Autodesk Fusion 360 part; units mm, degrees
(part 2 of 3)
  spline S416 degree 2 poles (1.0498, 18.6064) (0.9543, 18.5109) (0.9543, 18.3438) knots 0 0 0 1 1 1
  spline S417 degree 2 poles (1.3053, 18.7019) (1.1453, 18.7019) (1.0498, 18.6064) knots 0 0 0 1 1 1
  spline S418 degree 2 poles (1.5942, 18.5742) (1.4724, 18.7019) (1.3053, 18.7019) knots 0 0 0 1 1 1
  spline S419 degree 2 poles (1.7159, 18.2554) (1.7159, 18.4464) (1.5942, 18.5742) knots 0 0 0 1 1 1
  spline S420 degree 2 poles (1.704, 18.1289) (1.7159, 18.2101) (1.7159, 18.2554) knots 0 0 0 1 1 1
  line L121 (2.3987, 18.0788) -> (1.704, 18.1289)
  spline S421 degree 2 poles (2.3414, 18.3939) (2.3414, 18.2793) (2.3987, 18.0788) knots 0 0 0 1 1 1
  spline S422 degree 2 poles (2.4751, 18.7341) (2.3414, 18.6088) (2.3414, 18.3939) knots 0 0 0 1 1 1
  spline S423 degree 2 poles (2.8524, 18.8595) (2.6088, 18.8595) (2.4751, 18.7341) knots 0 0 0 1 1 1
  spline S424 degree 2 poles (3.2344, 18.7293) (3.0911, 18.8595) (2.8524, 18.8595) knots 0 0 0 1 1 1
  spline S425 degree 2 poles (3.3776, 18.4035) (3.3776, 18.5992) (3.2344, 18.7293) knots 0 0 0 1 1 1
  spline S426 degree 2 poles (3.2642, 18.0967) (3.3776, 18.2172) (3.3776, 18.4035) knots 0 0 0 1 1 1
  spline S427 degree 2 poles (2.8571, 17.9188) (3.1508, 17.9761) (3.2642, 18.0967) knots 0 0 0 1 1 1
  line L122 (2.9861, 16.9471) -> (2.8571, 17.9188)
  spline S428 degree 2 poles (3.5292, 17.2205) (3.3131, 17.0426) (2.9861, 16.9471) knots 0 0 0 1 1 1
  spline S429 degree 2 poles (3.8575, 17.6741) (3.7453, 17.3983) (3.5292, 17.2205) knots 0 0 0 1 1 1
  spline S430 degree 2 poles (3.9697, 18.4273) (3.9697, 17.9498) (3.8575, 17.6741) knots 0 0 0 1 1 1
  spline S431 degree 2 poles (3.8181, 19.2176) (3.9697, 18.9168) (3.9697, 18.4273) knots 0 0 0 1 1 1
  spline S432 degree 2 poles (3.386, 19.6783) (3.6665, 19.5184) (3.8181, 19.2176) knots 0 0 0 1 1 1
  spline S433 degree 2 poles (2.7998, 19.8383) (3.1054, 19.8383) (3.386, 19.6783) knots 0 0 0 1 1 1
  spline S434 degree 2 poles (2.3808, 19.7416) (2.5563, 19.8383) (2.7998, 19.8383) knots 0 0 0 1 1 1
  spline S435 degree 2 poles (2.0979, 19.4706) (2.2054, 19.6449) (2.3808, 19.7416) knots 0 0 0 1 1 1
  spline S436 degree 2 poles (1.9809, 19.1603) (2.0311, 19.3632) (2.0979, 19.4706) knots 0 0 0 1 1 1
  spline S437 degree 2 poles (1.6586, 19.5351) (1.8425, 19.411) (1.9809, 19.1603) knots 0 0 0 1 1 1
  spline S438 degree 2 poles (1.248, 19.6592) (1.4748, 19.6592) (1.6586, 19.5351) knots 0 0 0 1 1 1
  spline S439 degree 2 poles (0.6058, 19.3537) (0.8612, 19.6592) (1.248, 19.6592) knots 0 0 0 1 1 1
  spline S440 degree 2 poles (0.3503, 18.3629) (0.3503, 19.0481) (0.6058, 19.3537) knots 0 0 0 1 1 1
  spline S441 degree 2 poles (0.5843, 17.4401) (0.3503, 17.766) (0.3503, 18.3629) knots 0 0 0 1 1 1
  spline S442 degree 2 poles (1.2575, 16.9996) (0.8183, 17.1142) (0.5843, 17.4401) knots 0 0 0 1 1 1
  line L123 (1.4223, 17.9188) -> (1.2575, 16.9996)
  spline S443 degree 2 poles (1.0582, 18.0644) (1.162, 17.957) (1.4223, 17.9188) knots 0 0 0 1 1 1
  line L124 (6.5014, 21.9082) -> (6.5014, 20.9722)
  line L125 (6.5014, 20.9722) -> (5.3999, 21.9082)
  line L126 (5.3999, 21.9082) -> (6.5014, 21.9082)
  line L127 (7.91, 22.7558) -> (7.91, 21.9082)
  line L128 (7.2558, 22.7558) -> (7.91, 22.7558)
  line L129 (7.2558, 23.1951) -> (7.2558, 22.7558)
  line L130 (6.5014, 23.1951) -> (7.2558, 23.1951)
  line L131 (6.5014, 22.7558) -> (6.5014, 23.1951)
  line L132 (4.3503, 22.7558) -> (6.5014, 22.7558)
  line L133 (4.3503, 21.9082) -> (4.3503, 22.7558)
  line L134 (6.456, 20.1367) -> (4.3503, 21.9082)
  line L135 (7.2558, 20.1367) -> (6.456, 20.1367)
  line L136 (7.2558, 21.9082) -> (7.2558, 20.1367)
  line L137 (7.91, 21.9082) -> (7.2558, 21.9082)
  spline S444 degree 2 poles (2.1481, 21.2015) (1.4867, 21.2015) (1.242, 21.309) knots -1 -1 -1 0 0 0
  spline S445 degree 2 poles (1.242, 21.309) (0.9973, 21.4164) (0.9973, 21.6575) knots -1 -1 -1 0 0 0
  spline S446 degree 2 poles (0.9973, 21.6575) (0.9973, 21.8939) (1.2373, 22.0121) knots -1 -1 -1 0 0 0
  spline S447 degree 2 poles (1.2373, 22.0121) (1.4772, 22.1303) (2.1743, 22.1303) knots -1 -1 -1 0 0 0
  spline S448 degree 2 poles (2.1743, 22.1303) (2.6494, 22.1303) (2.8738, 22.0789) knots -1 -1 -1 0 0 0
  spline S449 degree 2 poles (2.8738, 22.0789) (3.0983, 22.0276) (3.2021, 21.919) knots -1 -1 -1 0 0 0
  spline S450 degree 2 poles (3.2021, 21.919) (3.306, 21.8103) (3.306, 21.6623) knots -1 -1 -1 0 0 0
  spline S451 degree 2 poles (3.306, 21.6623) (3.306, 21.4379) (3.0613, 21.3197) knots -1 -1 -1 0 0 0
  spline S452 degree 2 poles (3.0613, 21.3197) (2.8165, 21.2015) (2.1481, 21.2015) knots -1 -1 -1 0 0 0
  spline S453 degree 2 poles (3.4158, 20.5044) (3.2224, 20.3779) (2.887, 20.3074) knots 0 0 0 1 1 1
  spline S454 degree 2 poles (3.8288, 20.9509) (3.688, 20.6787) (3.4158, 20.5044) knots 0 0 0 1 1 1
  spline S455 degree 2 poles (3.9697, 21.6647) (3.9697, 21.223) (3.8288, 20.9509) knots 0 0 0 1 1 1
  spline S456 degree 2 poles (3.528, 22.7749) (3.9697, 22.4526) (3.9697, 21.6647) knots 0 0 0 1 1 1
  spline S457 degree 2 poles (2.1337, 23.0972) (3.0863, 23.0972) (3.528, 22.7749) knots 0 0 0 1 1 1
  spline S458 degree 2 poles (1.3172, 22.9993) (1.7088, 23.0972) (2.1337, 23.0972) knots 0 0 0 1 1 1
  spline S459 degree 2 poles (0.9579, 22.8668) (1.1119, 22.9492) (1.3172, 22.9993) knots 0 0 0 1 1 1
  spline S460 degree 2 poles (0.6643, 22.6412) (0.8039, 22.7844) (0.9579, 22.8668) knots 0 0 0 1 1 1
  spline S461 degree 2 poles (0.4375, 22.2711) (0.5246, 22.4979) (0.6643, 22.6412) knots 0 0 0 1 1 1
  spline S462 degree 2 poles (0.3503, 21.691) (0.3503, 22.0443) (0.4375, 22.2711) knots 0 0 0 1 1 1
  spline S463 degree 2 poles (0.749, 20.5963) (0.3503, 20.9556) (0.3503, 21.691) knots 0 0 0 1 1 1
  spline S464 degree 2 poles (2.1457, 20.237) (1.1477, 20.237) (0.749, 20.5963) knots 0 0 0 1 1 1
  spline S465 degree 2 poles (2.887, 20.3074) (2.5515, 20.237) (2.1457, 20.237) knots 0 0 0 1 1 1
  line L138 (-4.8826, 21.6074) -> (-4.8826, 23.1258)
  spline S466 degree 2 poles (-5.0951, 21.8402) (-5.0139, 21.7411) (-4.8826, 21.6074) knots 0 0 0 1 1 1
  spline S467 degree 2 poles (-5.3792, 22.2329) (-5.1763, 21.9393) (-5.0951, 21.8402) knots 0 0 0 1 1 1
  spline S468 degree 2 poles (-6.0191, 22.9145) (-5.7278, 22.7271) (-5.3792, 22.2329) knots 0 0 0 1 1 1
  spline S469 degree 2 poles (-6.6302, 23.1019) (-6.3103, 23.1019) (-6.0191, 22.9145) knots 0 0 0 1 1 1
  spline S470 degree 2 poles (-7.1734, 22.9384) (-6.9311, 23.1019) (-6.6302, 23.1019) knots 0 0 0 1 1 1
  spline S471 degree 2 poles (-7.5327, 22.4896) (-7.4157, 22.7749) (-7.1734, 22.9384) knots 0 0 0 1 1 1
  spline S472 degree 2 poles (-7.6497, 21.691) (-7.6497, 22.2043) (-7.5327, 22.4896) knots 0 0 0 1 1 1
  spline S473 degree 2 poles (-7.5267, 20.921) (-7.6497, 21.1992) (-7.6497, 21.691) knots 0 0 0 1 1 1
  spline S474 degree 2 poles (-7.1734, 20.4901) (-7.4038, 20.6429) (-7.5267, 20.921) knots 0 0 0 1 1 1
  spline S475 degree 2 poles (-6.5324, 20.28) (-6.943, 20.3373) (-7.1734, 20.4901) knots 0 0 0 1 1 1
  line L139 (-6.4536, 21.2541) -> (-6.5324, 20.28)
  spline S476 degree 2 poles (-6.8666, 21.4128) (-6.7496, 21.2947) (-6.4536, 21.2541) knots 0 0 0 1 1 1
  spline S477 degree 2 poles (-6.9836, 21.7172) (-6.9836, 21.531) (-6.8666, 21.4128) knots 0 0 0 1 1 1
  spline S478 degree 2 poles (-6.8702, 22.0145) (-6.9836, 21.8963) (-6.9836, 21.7172) knots 0 0 0 1 1 1
  spline S479 degree 2 poles (-6.5968, 22.1326) (-6.7568, 22.1326) (-6.8702, 22.0145) knots 0 0 0 1 1 1
  spline S480 degree 2 poles (-6.2841, 22.0133) (-6.4488, 22.1326) (-6.5968, 22.1326) knots 0 0 0 1 1 1
  spline S481 degree 2 poles (-5.8018, 21.4665) (-6.1193, 21.8939) (-6.2841, 22.0133) knots 0 0 0 1 1 1
  spline S482 degree 2 poles (-4.9029, 20.5128) (-5.2837, 20.767) (-5.8018, 21.4665) knots 0 0 0 1 1 1
  spline S483 degree 2 poles (-4.09, 20.2084) (-4.5221, 20.2585) (-4.9029, 20.5128) knots 0 0 0 1 1 1
  line L140 (-4.09, 23.1258) -> (-4.09, 20.2084)
  line L141 (-4.8826, 23.1258) -> (-4.09, 23.1258)
  line L142 (22.4107, 17.9021) -> (22.2913, 17.0736)
  spline S484 degree 2 poles (22.2292, 18.117) (22.2794, 18.0191) (22.4107, 17.9021) knots 0 0 0 1 1 1
  spline S485 degree 2 poles (22.16, 18.3891) (22.16, 18.2483) (22.2292, 18.117) knots 0 0 0 1 1 1
  spline S486 degree 2 poles (22.3056, 18.7449) (22.16, 18.6112) (22.16, 18.3891) knots 0 0 0 1 1 1
  spline S487 degree 2 poles (22.764, 18.8786) (22.4513, 18.8786) (22.3056, 18.7449) knots 0 0 0 1 1 1
  spline S488 degree 2 poles (23.2236, 18.746) (23.0696, 18.8786) (22.764, 18.8786) knots 0 0 0 1 1 1
  spline S489 degree 2 poles (23.3776, 18.4106) (23.3776, 18.6135) (23.2236, 18.746) knots 0 0 0 1 1 1
  spline S490 degree 2 poles (23.2546, 18.0979) (23.3776, 18.2292) (23.3776, 18.4106) knots 0 0 0 1 1 1
  spline S491 degree 2 poles (22.8953, 17.9307) (23.1317, 17.9665) (23.2546, 18.0979) knots 0 0 0 1 1 1
  line L143 (23.0028, 16.9471) -> (22.8953, 17.9307)
  spline S492 degree 2 poles (23.4134, 17.1262) (23.2487, 17.0187) (23.0028, 16.9471) knots 0 0 0 1 1 1
  spline S493 degree 2 poles (23.7083, 17.4067) (23.5781, 17.2336) (23.4134, 17.1262) knots 0 0 0 1 1 1
  spline S494 degree 2 poles (23.904, 17.8269) (23.8384, 17.5798) (23.7083, 17.4067) knots 0 0 0 1 1 1
  spline S495 degree 2 poles (23.9697, 18.4202) (23.9697, 18.074) (23.904, 17.8269) knots 0 0 0 1 1 1
  spline S496 degree 2 poles (23.805, 19.2116) (23.9697, 18.9024) (23.9697, 18.4202) knots 0 0 0 1 1 1
  spline S497 degree 2 poles (23.3275, 19.6891) (23.6402, 19.5208) (23.805, 19.2116) knots 0 0 0 1 1 1
  spline S498 degree 2 poles (22.6757, 19.8574) (23.0147, 19.8574) (23.3275, 19.6891) knots 0 0 0 1 1 1
  spline S499 degree 2 poles (21.8759, 19.5303) (22.1934, 19.8574) (22.6757, 19.8574) knots 0 0 0 1 1 1
  spline S500 degree 2 poles (21.5584, 18.678) (21.5584, 19.2032) (21.8759, 19.5303) knots 0 0 0 1 1 1
  spline S501 degree 2 poles (21.5966, 18.3641) (21.5584, 18.5228) (21.5584, 18.678) knots 0 0 0 1 1 1
  spline S502 degree 2 poles (21.7112, 18.0429) (21.6348, 18.2053) (21.5966, 18.3641) knots 0 0 0 1 1 1
  line L144 (21.1859, 18.1265) -> (21.7112, 18.0429)
  line L145 (21.1859, 19.6903) -> (21.1859, 18.1265)
  line L146 (20.41, 19.6903) -> (21.1859, 19.6903)
  line L147 (20.41, 17.3816) -> (20.41, 19.6903)
  line L148 (22.2913, 17.0736) -> (20.41, 17.3816)
  line L149 (18.5014, 18.7186) -> (18.5014, 17.7826)
  line L150 (18.5014, 17.7826) -> (17.3999, 18.7186)
  line L151 (17.3999, 18.7186) -> (18.5014, 18.7186)
  line L152 (19.91, 19.5661) -> (19.91, 18.7186)
  line L153 (19.2558, 19.5661) -> (19.91, 19.5661)
  line L154 (19.2558, 20.0054) -> (19.2558, 19.5661)
  line L155 (18.5014, 20.0054) -> (19.2558, 20.0054)
  line L156 (18.5014, 19.5661) -> (18.5014, 20.0054)
  line L157 (16.3503, 19.5661) -> (18.5014, 19.5661)
  line L158 (16.3503, 18.7186) -> (16.3503, 19.5661)
  line L159 (18.456, 16.9471) -> (16.3503, 18.7186)
  line L160 (19.2558, 16.9471) -> (18.456, 16.9471)
  line L161 (19.2558, 18.7186) -> (19.2558, 16.9471)
  line L162 (19.91, 18.7186) -> (19.2558, 18.7186)
  spline S503 degree 2 poles (-11.0958, 17.7183) (-11.3202, 17.9928) (-11.6497, 18.148) knots 0 0 0 1 1 1
  spline S504 degree 2 poles (-10.7114, 16.9471) (-10.8714, 17.4437) (-11.0958, 17.7183) knots 0 0 0 1 1 1
  line L163 (-9.914, 16.9471) -> (-10.7114, 16.9471)
  spline S505 degree 2 poles (-10.1289, 17.507) (-10.0167, 17.2837) (-9.914, 16.9471) knots 0 0 0 1 1 1
  spline S506 degree 2 poles (-10.4225, 17.9689) (-10.2411, 17.7302) (-10.1289, 17.507) knots 0 0 0 1 1 1
  line L164 (-8.09, 17.9689) -> (-10.4225, 17.9689)
  line L165 (-8.09, 18.9526) -> (-8.09, 17.9689)
  line L166 (-11.6497, 18.9526) -> (-8.09, 18.9526)
  line L167 (-11.6497, 18.148) -> (-11.6497, 18.9526)
  spline S507 degree 2 poles (-9.1524, 20.9795) (-9.3959, 20.9795) (-9.5392, 21.1144) knots -1 -1 -1 0 0 0
  spline S508 degree 2 poles (-9.5392, 21.1144) (-9.6824, 21.2493) (-9.6824, 21.4307) knots -1 -1 -1 0 0 0
  spline S509 degree 2 poles (-9.6824, 21.4307) (-9.6824, 21.6146) (-9.5344, 21.7542) knots -1 -1 -1 0 0 0
  spline S510 degree 2 poles (-9.5344, 21.7542) (-9.3864, 21.8939) (-9.1548, 21.8939) knots -1 -1 -1 0 0 0
  spline S511 degree 2 poles (-9.1548, 21.8939) (-8.9256, 21.8939) (-8.7764, 21.7554) knots -1 -1 -1 0 0 0
  spline S512 degree 2 poles (-8.7764, 21.7554) (-8.6272, 21.617) (-8.6272, 21.4427) knots -1 -1 -1 0 0 0
  spline S513 degree 2 poles (-8.6272, 21.4427) (-8.6272, 21.2612) (-8.774, 21.1204) knots -1 -1 -1 0 0 0
  spline S514 degree 2 poles (-8.774, 21.1204) (-8.9208, 20.9795) (-9.1524, 20.9795) knots -1 -1 -1 0 0 0
  spline S515 degree 2 poles (-10.6589, 21.032) (-10.8356, 21.032) (-10.9466, 21.143) knots -1 -1 -1 0 0 0
  spline S516 degree 2 poles (-10.9466, 21.143) (-11.0576, 21.2541) (-11.0576, 21.4307) knots -1 -1 -1 0 0 0
  spline S517 degree 2 poles (-11.0576, 21.4307) (-11.0576, 21.605) (-10.9442, 21.7172) knots -1 -1 -1 0 0 0
  spline S518 degree 2 poles (-10.9442, 21.7172) (-10.8308, 21.8294) (-10.6493, 21.8294) knots -1 -1 -1 0 0 0
  spline S519 degree 2 poles (-10.6493, 21.8294) (-10.4751, 21.8294) (-10.3652, 21.722) knots -1 -1 -1 0 0 0
  spline S520 degree 2 poles (-10.3652, 21.722) (-10.2554, 21.6146) (-10.2554, 21.4474) knots -1 -1 -1 0 0 0
  spline S521 degree 2 poles (-10.2554, 21.4474) (-10.2554, 21.2588) (-10.3664, 21.1454) knots -1 -1 -1 0 0 0
  spline S522 degree 2 poles (-10.3664, 21.1454) (-10.4774, 21.032) (-10.6589, 21.032) knots -1 -1 -1 0 0 0
  spline S523 degree 2 poles (-9.119, 20.0102) (-9.427, 20.0102) (-9.6406, 20.1535) knots 0 0 0 1 1 1
  spline S524 degree 2 poles (-8.5484, 20.163) (-8.8038, 20.0102) (-9.119, 20.0102) knots 0 0 0 1 1 1
  spline S525 degree 2 poles (-8.1616, 20.6095) (-8.2929, 20.3158) (-8.5484, 20.163) knots 0 0 0 1 1 1
  spline S526 degree 2 poles (-8.0303, 21.4594) (-8.0303, 20.9031) (-8.1616, 20.6095) knots 0 0 0 1 1 1
  spline S527 degree 2 poles (-8.0888, 22.0169) (-8.0303, 21.7554) (-8.0303, 21.4594) knots 0 0 0 1 1 1
  spline S528 degree 2 poles (-8.2714, 22.4538) (-8.1473, 22.2783) (-8.0888, 22.0169) knots 0 0 0 1 1 1
  spline S529 degree 2 poles (-8.6236, 22.7498) (-8.3956, 22.6292) (-8.2714, 22.4538) knots 0 0 0 1 1 1
  spline S530 degree 2 poles (-9.1142, 22.8704) (-8.8516, 22.8704) (-8.6236, 22.7498) knots 0 0 0 1 1 1
  spline S531 degree 2 poles (-9.6108, 22.7307) (-9.3864, 22.8704) (-9.1142, 22.8704) knots 0 0 0 1 1 1
  spline S532 degree 2 poles (-9.9713, 22.3069) (-9.8352, 22.591) (-9.6108, 22.7307) knots 0 0 0 1 1 1
  spline S533 degree 2 poles (-10.2674, 22.6221) (-10.1146, 22.5218) (-9.9713, 22.3069) knots 0 0 0 1 1 1
  spline S534 degree 2 poles (-10.709, 22.7558) (-10.4727, 22.7558) (-10.2674, 22.6221) knots 0 0 0 1 1 1
  spline S535 degree 2 poles (-11.3823, 22.4203) (-11.1149, 22.7558) (-10.709, 22.7558) knots 0 0 0 1 1 1
  spline S536 degree 2 poles (-11.6497, 21.383) (-11.6497, 22.0849) (-11.3823, 22.4203) knots 0 0 0 1 1 1
  spline S537 degree 2 poles (-11.4348, 20.5307) (-11.6497, 20.853) (-11.6497, 21.383) knots 0 0 0 1 1 1
  spline S538 degree 2 poles (-10.7162, 20.1176) (-11.1555, 20.1176) (-11.4348, 20.5307) knots 0 0 0 1 1 1
  spline S539 degree 2 poles (-10.2435, 20.2609) (-10.4488, 20.1176) (-10.7162, 20.1176) knots 0 0 0 1 1 1
  spline S540 degree 2 poles (-9.9713, 20.5951) (-10.0931, 20.3659) (-10.2435, 20.2609) knots 0 0 0 1 1 1
  spline S541 degree 2 poles (-9.6406, 20.1535) (-9.8543, 20.2967) (-9.9713, 20.5951) knots 0 0 0 1 1 1
  spline S542 degree 2 poles (-17.8519, 20.9747) (-18.5133, 20.9747) (-18.758, 21.0822) knots -1 -1 -1 0 0 0
  spline S543 degree 2 poles (-18.758, 21.0822) (-19.0027, 21.1896) (-19.0027, 21.4307) knots -1 -1 -1 0 0 0
  spline S544 degree 2 poles (-19.0027, 21.4307) (-19.0027, 21.6671) (-18.7627, 21.7853) knots -1 -1 -1 0 0 0
  spline S545 degree 2 poles (-18.7627, 21.7853) (-18.5228, 21.9035) (-17.8257, 21.9035) knots -1 -1 -1 0 0 0
  spline S546 degree 2 poles (-17.8257, 21.9035) (-17.3506, 21.9035) (-17.1262, 21.8521) knots -1 -1 -1 0 0 0
  spline S547 degree 2 poles (-17.1262, 21.8521) (-16.9017, 21.8008) (-16.7979, 21.6922) knots -1 -1 -1 0 0 0
  spline S548 degree 2 poles (-16.7979, 21.6922) (-16.694, 21.5835) (-16.694, 21.4355) knots -1 -1 -1 0 0 0
  spline S549 degree 2 poles (-16.694, 21.4355) (-16.694, 21.2111) (-16.9387, 21.0929) knots -1 -1 -1 0 0 0
  spline S550 degree 2 poles (-16.9387, 21.0929) (-17.1835, 20.9747) (-17.8519, 20.9747) knots -1 -1 -1 0 0 0
  spline S551 degree 2 poles (-16.5842, 20.2776) (-16.7776, 20.1511) (-17.113, 20.0806) knots 0 0 0 1 1 1
  spline S552 degree 2 poles (-16.1712, 20.7241) (-16.312, 20.4519) (-16.5842, 20.2776) knots 0 0 0 1 1 1
  spline S553 degree 2 poles (-16.0303, 21.4379) (-16.0303, 20.9962) (-16.1712, 20.7241) knots 0 0 0 1 1 1
  spline S554 degree 2 poles (-16.472, 22.5481) (-16.0303, 22.2258) (-16.0303, 21.4379) knots 0 0 0 1 1 1
  spline S555 degree 2 poles (-17.8663, 22.8704) (-16.9137, 22.8704) (-16.472, 22.5481) knots 0 0 0 1 1 1
  spline S556 degree 2 poles (-18.6828, 22.7725) (-18.2912, 22.8704) (-17.8663, 22.8704) knots 0 0 0 1 1 1
  spline S557 degree 2 poles (-19.0421, 22.64) (-18.8881, 22.7223) (-18.6828, 22.7725) knots 0 0 0 1 1 1
  spline S558 degree 2 poles (-19.3357, 22.4144) (-19.1961, 22.5576) (-19.0421, 22.64) knots 0 0 0 1 1 1
  spline S559 degree 2 poles (-19.5625, 22.0443) (-19.4754, 22.2711) (-19.3357, 22.4144) knots 0 0 0 1 1 1
  spline S560 degree 2 poles (-19.6497, 21.4642) (-19.6497, 21.8175) (-19.5625, 22.0443) knots 0 0 0 1 1 1
  spline S561 degree 2 poles (-19.251, 20.3695) (-19.6497, 20.7288) (-19.6497, 21.4642) knots 0 0 0 1 1 1
  spline S562 degree 2 poles (-17.8543, 20.0102) (-18.8523, 20.0102) (-19.251, 20.3695) knots 0 0 0 1 1 1
  spline S563 degree 2 poles (-17.113, 20.0806) (-17.4485, 20.0102) (-17.8543, 20.0102) knots 0 0 0 1 1 1
  line L168 (-4.8826, 18.3462) -> (-4.8826, 19.8646)
  spline S564 degree 2 poles (-5.0951, 18.5789) (-5.0139, 18.4798) (-4.8826, 18.3462) knots 0 0 0 1 1 1
  spline S565 degree 2 poles (-5.3792, 18.9717) (-5.1763, 18.678) (-5.0951, 18.5789) knots 0 0 0 1 1 1
  spline S566 degree 2 poles (-6.0191, 19.6533) (-5.7278, 19.4659) (-5.3792, 18.9717) knots 0 0 0 1 1 1
  spline S567 degree 2 poles (-6.6302, 19.8407) (-6.3103, 19.8407) (-6.0191, 19.6533) knots 0 0 0 1 1 1
  spline S568 degree 2 poles (-7.1734, 19.6772) (-6.9311, 19.8407) (-6.6302, 19.8407) knots 0 0 0 1 1 1
  spline S569 degree 2 poles (-7.5327, 19.2283) (-7.4157, 19.5136) (-7.1734, 19.6772) knots 0 0 0 1 1 1
  spline S570 degree 2 poles (-7.6497, 18.4297) (-7.6497, 18.943) (-7.5327, 19.2283) knots 0 0 0 1 1 1
  spline S571 degree 2 poles (-7.5267, 17.6598) (-7.6497, 17.9379) (-7.6497, 18.4297) knots 0 0 0 1 1 1
  spline S572 degree 2 poles (-7.1734, 17.2288) (-7.4038, 17.3816) (-7.5267, 17.6598) knots 0 0 0 1 1 1
  spline S573 degree 2 poles (-6.5324, 17.0187) (-6.943, 17.076) (-7.1734, 17.2288) knots 0 0 0 1 1 1
  line L169 (-6.4536, 17.9928) -> (-6.5324, 17.0187)
  spline S574 degree 2 poles (-6.8666, 18.1516) (-6.7496, 18.0334) (-6.4536, 17.9928) knots 0 0 0 1 1 1
  spline S575 degree 2 poles (-6.9836, 18.456) (-6.9836, 18.2698) (-6.8666, 18.1516) knots 0 0 0 1 1 1
  spline S576 degree 2 poles (-6.8702, 18.7532) (-6.9836, 18.635) (-6.9836, 18.456) knots 0 0 0 1 1 1
  spline S577 degree 2 poles (-6.5968, 18.8714) (-6.7568, 18.8714) (-6.8702, 18.7532) knots 0 0 0 1 1 1
  spline S578 degree 2 poles (-6.2841, 18.752) (-6.4488, 18.8714) (-6.5968, 18.8714) knots 0 0 0 1 1 1
  spline S579 degree 2 poles (-5.8018, 18.2053) (-6.1193, 18.6326) (-6.2841, 18.752) knots 0 0 0 1 1 1
  spline S580 degree 2 poles (-4.9029, 17.2515) (-5.2837, 17.5058) (-5.8018, 18.2053) knots 0 0 0 1 1 1
  spline S581 degree 2 poles (-4.09, 16.9471) (-4.5221, 16.9972) (-4.9029, 17.2515) knots 0 0 0 1 1 1
  line L170 (-4.09, 19.8646) -> (-4.09, 16.9471)
  line L171 (-4.8826, 19.8646) -> (-4.09, 19.8646)
  line L172 (-23.4986, -8.6639) -> (-23.4986, -9.6)
  line L173 (-23.4986, -9.6) -> (-24.6001, -8.6639)
  line L174 (-24.6001, -8.6639) -> (-23.4986, -8.6639)
  line L175 (-22.09, -7.8164) -> (-22.09, -8.6639)
  line L176 (-22.7442, -7.8164) -> (-22.09, -7.8164)
  line L177 (-22.7442, -7.3771) -> (-22.7442, -7.8164)
  line L178 (-23.4986, -7.3771) -> (-22.7442, -7.3771)
  line L179 (-23.4986, -7.8164) -> (-23.4986, -7.3771)
  line L180 (-25.6497, -7.8164) -> (-23.4986, -7.8164)
  line L181 (-25.6497, -8.6639) -> (-25.6497, -7.8164)
  line L182 (-23.544, -10.4354) -> (-25.6497, -8.6639)
  line L183 (-22.7442, -10.4354) -> (-23.544, -10.4354)
  line L184 (-22.7442, -8.6639) -> (-22.7442, -10.4354)
  line L185 (-22.09, -8.6639) -> (-22.7442, -8.6639)
  spline S582 degree 2 poles (8.7569, -9.2417) (8.4775, -9.2417) (8.3271, -9.1044) knots -1 -1 -1 0 0 0
  spline S583 degree 2 poles (8.3271, -9.1044) (8.1767, -8.9671) (8.1767, -8.7642) knots -1 -1 -1 0 0 0
  spline S584 degree 2 poles (8.1767, -8.7642) (8.1767, -8.5661) (8.3319, -8.4324) knots -1 -1 -1 0 0 0
  spline S585 degree 2 poles (8.3319, -8.4324) (8.4871, -8.2987) (8.7831, -8.2987) knots -1 -1 -1 0 0 0
  spline S586 degree 2 poles (8.7831, -8.2987) (9.072, -8.2987) (9.2176, -8.4276) knots -1 -1 -1 0 0 0
  spline S587 degree 2 poles (9.2176, -8.4276) (9.3633, -8.5565) (9.3633, -8.7475) knots -1 -1 -1 0 0 0
  spline S588 degree 2 poles (9.3633, -8.7475) (9.3633, -8.9552) (9.2021, -9.0985) knots -1 -1 -1 0 0 0
  spline S589 degree 2 poles (9.2021, -9.0985) (9.041, -9.2417) (8.7569, -9.2417) knots -1 -1 -1 0 0 0
  spline S590 degree 2 poles (6.447, -8.0969) (6.5437, -7.8546) (6.7299, -7.6946) knots 0 0 0 1 1 1
  spline S591 degree 2 poles (6.3503, -8.7571) (6.3503, -8.3392) (6.447, -8.0969) knots 0 0 0 1 1 1
  spline S592 degree 2 poles (6.7908, -9.8624) (6.3503, -9.4637) (6.3503, -8.7571) knots 0 0 0 1 1 1
  spline S593 degree 2 poles (8.1791, -10.2611) (7.2313, -10.2611) (6.7908, -9.8624) knots 0 0 0 1 1 1
  spline S594 degree 2 poles (9.2188, -10.0713) (8.8261, -10.2611) (8.1791, -10.2611) knots 0 0 0 1 1 1
  spline S595 degree 2 poles (9.7906, -9.564) (9.6116, -9.8815) (9.2188, -10.0713) knots 0 0 0 1 1 1
  spline S596 degree 2 poles (9.9697, -8.7212) (9.9697, -9.2465) (9.7906, -9.564) knots 0 0 0 1 1 1
  spline S597 degree 2 poles (9.8229, -7.9943) (9.9697, -8.2843) (9.9697, -8.7212) knots 0 0 0 1 1 1
  spline S598 degree 2 poles (9.3895, -7.5406) (9.676, -7.7042) (9.8229, -7.9943) knots 0 0 0 1 1 1
  spline S599 degree 2 poles (8.7569, -7.3771) (9.103, -7.3771) (9.3895, -7.5406) knots 0 0 0 1 1 1
  spline S600 degree 2 poles (7.9093, -7.7006) (8.2436, -7.3771) (8.7569, -7.3771) knots 0 0 0 1 1 1
  spline S601 degree 2 poles (7.5751, -8.492) (7.5751, -8.0241) (7.9093, -7.7006) knots 0 0 0 1 1 1
  spline S602 degree 2 poles (7.6598, -8.917) (7.5751, -8.7332) (7.5751, -8.492) knots 0 0 0 1 1 1
  spline S603 degree 2 poles (7.9213, -9.2751) (7.7446, -9.1008) (7.6598, -8.917) knots 0 0 0 1 1 1
  spline S604 degree 2 poles (7.1859, -9.1343) (7.3578, -9.2298) (7.9213, -9.2751) knots 0 0 0 1 1 1
  spline S605 degree 2 poles (6.9472, -8.7666) (6.9472, -9.003) (7.1859, -9.1343) knots 0 0 0 1 1 1
  spline S606 degree 2 poles (7.0307, -8.5458) (6.9472, -8.6353) (6.9472, -8.7666) knots 0 0 0 1 1 1
  spline S607 degree 2 poles (7.3172, -8.418) (7.1143, -8.4562) (7.0307, -8.5458) knots 0 0 0 1 1 1
  line L186 (7.1979, -7.4511) -> (7.3172, -8.418)
  spline S608 degree 2 poles (6.7299, -7.6946) (6.9161, -7.5347) (7.1979, -7.4511) knots 0 0 0 1 1 1
  line L187 (-2.8826, -12.269) -> (-2.8826, -10.7506)
  spline S609 degree 2 poles (-3.0951, -12.0362) (-3.0139, -12.1353) (-2.8826, -12.269) knots 0 0 0 1 1 1
  spline S610 degree 2 poles (-3.3792, -11.6435) (-3.1763, -11.9371) (-3.0951, -12.0362) knots 0 0 0 1 1 1
  spline S611 degree 2 poles (-4.0191, -10.9619) (-3.7278, -11.1493) (-3.3792, -11.6435) knots 0 0 0 1 1 1
  spline S612 degree 2 poles (-4.6302, -10.7744) (-4.3103, -10.7744) (-4.0191, -10.9619) knots 0 0 0 1 1 1
  spline S613 degree 2 poles (-5.1734, -10.938) (-4.9311, -10.7744) (-4.6302, -10.7744) knots 0 0 0 1 1 1
  spline S614 degree 2 poles (-5.5327, -11.3868) (-5.4157, -11.1015) (-5.1734, -10.938) knots 0 0 0 1 1 1
  spline S615 degree 2 poles (-5.6497, -12.1854) (-5.6497, -11.6721) (-5.5327, -11.3868) knots 0 0 0 1 1 1
  spline S616 degree 2 poles (-5.5267, -12.9554) (-5.6497, -12.6772) (-5.6497, -12.1854) knots 0 0 0 1 1 1
  spline S617 degree 2 poles (-5.1734, -13.3863) (-5.4038, -13.2335) (-5.5267, -12.9554) knots 0 0 0 1 1 1
  spline S618 degree 2 poles (-4.5324, -13.5964) (-4.943, -13.5391) (-5.1734, -13.3863) knots 0 0 0 1 1 1
  line L188 (-4.4536, -12.6223) -> (-4.5324, -13.5964)
  spline S619 degree 2 poles (-4.8666, -12.4636) (-4.7496, -12.5817) (-4.4536, -12.6223) knots 0 0 0 1 1 1
  spline S620 degree 2 poles (-4.9836, -12.1592) (-4.9836, -12.3454) (-4.8666, -12.4636) knots 0 0 0 1 1 1
  spline S621 degree 2 poles (-4.8702, -11.8619) (-4.9836, -11.9801) (-4.9836, -12.1592) knots 0 0 0 1 1 1
  spline S622 degree 2 poles (-4.5968, -11.7438) (-4.7568, -11.7438) (-4.8702, -11.8619) knots 0 0 0 1 1 1
  spline S623 degree 2 poles (-4.2841, -11.8631) (-4.4488, -11.7438) (-4.5968, -11.7438) knots 0 0 0 1 1 1
  spline S624 degree 2 poles (-3.8018, -12.4098) (-4.1193, -11.9825) (-4.2841, -11.8631) knots 0 0 0 1 1 1
  spline S625 degree 2 poles (-2.9029, -13.3636) (-3.2837, -13.1094) (-3.8018, -12.4098) knots 0 0 0 1 1 1
  spline S626 degree 2 poles (-2.09, -13.668) (-2.5221, -13.6179) (-2.9029, -13.3636) knots 0 0 0 1 1 1
  line L189 (-2.09, -10.7506) -> (-2.09, -13.668)
  line L190 (-2.8826, -10.7506) -> (-2.09, -10.7506)
  spline S627 degree 2 poles (-11.2431, -9.2417) (-11.5225, -9.2417) (-11.6729, -9.1044) knots -1 -1 -1 0 0 0
  spline S628 degree 2 poles (-11.6729, -9.1044) (-11.8233, -8.9671) (-11.8233, -8.7642) knots -1 -1 -1 0 0 0
  spline S629 degree 2 poles (-11.8233, -8.7642) (-11.8233, -8.5661) (-11.6681, -8.4324) knots -1 -1 -1 0 0 0
  spline S630 degree 2 poles (-11.6681, -8.4324) (-11.5129, -8.2987) (-11.2169, -8.2987) knots -1 -1 -1 0 0 0
  spline S631 degree 2 poles (-11.2169, -8.2987) (-10.928, -8.2987) (-10.7824, -8.4276) knots -1 -1 -1 0 0 0
  spline S632 degree 2 poles (-10.7824, -8.4276) (-10.6367, -8.5565) (-10.6367, -8.7475) knots -1 -1 -1 0 0 0
  spline S633 degree 2 poles (-10.6367, -8.7475) (-10.6367, -8.9552) (-10.7979, -9.0985) knots -1 -1 -1 0 0 0
  spline S634 degree 2 poles (-10.7979, -9.0985) (-10.959, -9.2417) (-11.2431, -9.2417) knots -1 -1 -1 0 0 0
  spline S635 degree 2 poles (-13.553, -8.0969) (-13.4563, -7.8546) (-13.2701, -7.6946) knots 0 0 0 1 1 1
  spline S636 degree 2 poles (-13.6497, -8.7571) (-13.6497, -8.3392) (-13.553, -8.0969) knots 0 0 0 1 1 1
  spline S637 degree 2 poles (-13.2092, -9.8624) (-13.6497, -9.4637) (-13.6497, -8.7571) knots 0 0 0 1 1 1
  spline S638 degree 2 poles (-11.8209, -10.2611) (-12.7687, -10.2611) (-13.2092, -9.8624) knots 0 0 0 1 1 1
  spline S639 degree 2 poles (-10.7812, -10.0713) (-11.1739, -10.2611) (-11.8209, -10.2611) knots 0 0 0 1 1 1
  spline S640 degree 2 poles (-10.2094, -9.564) (-10.3884, -9.8815) (-10.7812, -10.0713) knots 0 0 0 1 1 1
  spline S641 degree 2 poles (-10.0303, -8.7212) (-10.0303, -9.2465) (-10.2094, -9.564) knots 0 0 0 1 1 1
  spline S642 degree 2 poles (-10.1771, -7.9943) (-10.0303, -8.2843) (-10.0303, -8.7212) knots 0 0 0 1 1 1
  spline S643 degree 2 poles (-10.6105, -7.5406) (-10.324, -7.7042) (-10.1771, -7.9943) knots 0 0 0 1 1 1
  spline S644 degree 2 poles (-11.2431, -7.3771) (-10.897, -7.3771) (-10.6105, -7.5406) knots 0 0 0 1 1 1
  spline S645 degree 2 poles (-12.0907, -7.7006) (-11.7564, -7.3771) (-11.2431, -7.3771) knots 0 0 0 1 1 1
  spline S646 degree 2 poles (-12.4249, -8.492) (-12.4249, -8.0241) (-12.0907, -7.7006) knots 0 0 0 1 1 1
  spline S647 degree 2 poles (-12.3402, -8.917) (-12.4249, -8.7332) (-12.4249, -8.492) knots 0 0 0 1 1 1
  spline S648 degree 2 poles (-12.0787, -9.2751) (-12.2554, -9.1008) (-12.3402, -8.917) knots 0 0 0 1 1 1
  spline S649 degree 2 poles (-12.8141, -9.1343) (-12.6422, -9.2298) (-12.0787, -9.2751) knots 0 0 0 1 1 1
  spline S650 degree 2 poles (-13.0528, -8.7666) (-13.0528, -9.003) (-12.8141, -9.1343) knots 0 0 0 1 1 1
  spline S651 degree 2 poles (-12.9693, -8.5458) (-13.0528, -8.6353) (-13.0528, -8.7666) knots 0 0 0 1 1 1
  spline S652 degree 2 poles (-12.6828, -8.418) (-12.8857, -8.4562) (-12.9693, -8.5458) knots 0 0 0 1 1 1
  line L191 (-12.8021, -7.4511) -> (-12.6828, -8.418)
  spline S653 degree 2 poles (-13.2701, -7.6946) (-13.0839, -7.5347) (-12.8021, -7.4511) knots 0 0 0 1 1 1
  spline S654 degree 2 poles (-0.6589, -9.2154) (-0.8356, -9.2154) (-0.9466, -9.1044) knots -1 -1 -1 0 0 0
  spline S655 degree 2 poles (-0.9466, -9.1044) (-1.0576, -8.9934) (-1.0576, -8.8167) knots -1 -1 -1 0 0 0
  spline S656 degree 2 poles (-1.0576, -8.8167) (-1.0576, -8.6425) (-0.9442, -8.5302) knots -1 -1 -1 0 0 0
  spline S657 degree 2 poles (-0.9442, -8.5302) (-0.8308, -8.418) (-0.6493, -8.418) knots -1 -1 -1 0 0 0
  spline S658 degree 2 poles (-0.6493, -8.418) (-0.4751, -8.418) (-0.3652, -8.5255) knots -1 -1 -1 0 0 0
  spline S659 degree 2 poles (-0.3652, -8.5255) (-0.2554, -8.6329) (-0.2554, -8.8) knots -1 -1 -1 0 0 0
  spline S660 degree 2 poles (-0.2554, -8.8) (-0.2554, -8.9886) (-0.3664, -9.102) knots -1 -1 -1 0 0 0
  spline S661 degree 2 poles (-0.3664, -9.102) (-0.4774, -9.2154) (-0.6589, -9.2154) knots -1 -1 -1 0 0 0
  spline S662 degree 2 poles (0.8476, -9.268) (0.6041, -9.268) (0.4608, -9.1331) knots -1 -1 -1 0 0 0
  spline S663 degree 2 poles (0.4608, -9.1331) (0.3176, -8.9982) (0.3176, -8.8167) knots -1 -1 -1 0 0 0
  spline S664 degree 2 poles (0.3176, -8.8167) (0.3176, -8.6329) (0.4656, -8.4932) knots -1 -1 -1 0 0 0
  spline S665 degree 2 poles (0.4656, -8.4932) (0.6136, -8.3536) (0.8452, -8.3536) knots -1 -1 -1 0 0 0
  spline S666 degree 2 poles (0.8452, -8.3536) (1.0744, -8.3536) (1.2236, -8.492) knots -1 -1 -1 0 0 0
  spline S667 degree 2 poles (1.2236, -8.492) (1.3728, -8.6305) (1.3728, -8.8048) knots -1 -1 -1 0 0 0
  spline S668 degree 2 poles (1.3728, -8.8048) (1.3728, -8.9862) (1.226, -9.1271) knots -1 -1 -1 0 0 0
  spline S669 degree 2 poles (1.226, -9.1271) (1.0792, -9.268) (0.8476, -9.268) knots -1 -1 -1 0 0 0
  spline S670 degree 2 poles (0.881, -10.2373) (0.573, -10.2373) (0.3594, -10.094) knots 0 0 0 1 1 1
  spline S671 degree 2 poles (1.4516, -10.0845) (1.1962, -10.2373) (0.881, -10.2373) knots 0 0 0 1 1 1
  spline S672 degree 2 poles (1.8384, -9.638) (1.7071, -9.9317) (1.4516, -10.0845) knots 0 0 0 1 1 1
  spline S673 degree 2 poles (1.9697, -8.7881) (1.9697, -9.3444) (1.8384, -9.638) knots 0 0 0 1 1 1
  spline S674 degree 2 poles (1.9112, -8.2306) (1.9697, -8.492) (1.9697, -8.7881) knots 0 0 0 1 1 1
  spline S675 degree 2 poles (1.7286, -7.7937) (1.8527, -7.9692) (1.9112, -8.2306) knots 0 0 0 1 1 1
  spline S676 degree 2 poles (1.3764, -7.4977) (1.6044, -7.6182) (1.7286, -7.7937) knots 0 0 0 1 1 1
  spline S677 degree 2 poles (0.8858, -7.3771) (1.1484, -7.3771) (1.3764, -7.4977) knots 0 0 0 1 1 1
  spline S678 degree 2 poles (0.3892, -7.5168) (0.6136, -7.3771) (0.8858, -7.3771) knots 0 0 0 1 1 1
  spline S679 degree 2 poles (0.0287, -7.9405) (0.1648, -7.6564) (0.3892, -7.5168) knots 0 0 0 1 1 1
  spline S680 degree 2 poles (-0.2674, -7.6254) (-0.1146, -7.7257) (0.0287, -7.9405) knots 0 0 0 1 1 1
  spline S681 degree 2 poles (-0.709, -7.4917) (-0.4727, -7.4917) (-0.2674, -7.6254) knots 0 0 0 1 1 1
  spline S682 degree 2 poles (-1.3823, -7.8271) (-1.1149, -7.4917) (-0.709, -7.4917) knots 0 0 0 1 1 1
  spline S683 degree 2 poles (-1.6497, -8.8645) (-1.6497, -8.1626) (-1.3823, -7.8271) knots 0 0 0 1 1 1
  spline S684 degree 2 poles (-1.4348, -9.7168) (-1.6497, -9.3945) (-1.6497, -8.8645) knots 0 0 0 1 1 1
  spline S685 degree 2 poles (-0.7162, -10.1298) (-1.1555, -10.1298) (-1.4348, -9.7168) knots 0 0 0 1 1 1
  spline S686 degree 2 poles (-0.2435, -9.9866) (-0.4488, -10.1298) (-0.7162, -10.1298) knots 0 0 0 1 1 1
  spline S687 degree 2 poles (0.0287, -9.6523) (-0.0931, -9.8815) (-0.2435, -9.9866) knots 0 0 0 1 1 1
  spline S688 degree 2 poles (0.3594, -10.094) (0.1457, -9.9508) (0.0287, -9.6523) knots 0 0 0 1 1 1
  line L192 (12.5014, -11.8273) -> (12.5014, -12.7633)
  line L193 (12.5014, -12.7633) -> (11.3999, -11.8273)
  line L194 (11.3999, -11.8273) -> (12.5014, -11.8273)
  line L195 (13.91, -10.9798) -> (13.91, -11.8273)
  line L196 (13.2558, -10.9798) -> (13.91, -10.9798)
  line L197 (13.2558, -10.5405) -> (13.2558, -10.9798)
  line L198 (12.5014, -10.5405) -> (13.2558, -10.5405)
  line L199 (12.5014, -10.9798) -> (12.5014, -10.5405)
  line L200 (10.3503, -10.9798) -> (12.5014, -10.9798)
  line L201 (10.3503, -11.8273) -> (10.3503, -10.9798)
  line L202 (12.456, -13.5988) -> (10.3503, -11.8273)
  line L203 (13.2558, -13.5988) -> (12.456, -13.5988)
  line L204 (13.2558, -11.8273) -> (13.2558, -13.5988)
  line L205 (13.91, -11.8273) -> (13.2558, -11.8273)
  spline S689 degree 2 poles (-17.0958, -12.5149) (-17.3202, -12.2403) (-17.6497, -12.0852) knots 0 0 0 1 1 1
  spline S690 degree 2 poles (-16.7114, -13.286) (-16.8714, -12.7895) (-17.0958, -12.5149) knots 0 0 0 1 1 1
  line L206 (-15.914, -13.286) -> (-16.7114, -13.286)
  spline S691 degree 2 poles (-16.1289, -12.7262) (-16.0167, -12.9494) (-15.914, -13.286) knots 0 0 0 1 1 1
  spline S692 degree 2 poles (-16.4225, -12.2642) (-16.2411, -12.503) (-16.1289, -12.7262) knots 0 0 0 1 1 1
  line L207 (-14.09, -12.2642) -> (-16.4225, -12.2642)
  line L208 (-14.09, -11.2806) -> (-14.09, -12.2642)
  line L209 (-17.6497, -11.2806) -> (-14.09, -11.2806)
  line L210 (-17.6497, -12.0852) -> (-17.6497, -11.2806)
  spline S693 degree 2 poles (12.1481, -9.2727) (11.4867, -9.2727) (11.242, -9.1653) knots -1 -1 -1 0 0 0
  spline S694 degree 2 poles (11.242, -9.1653) (10.9973, -9.0579) (10.9973, -8.8167) knots -1 -1 -1 0 0 0
  spline S695 degree 2 poles (10.9973, -8.8167) (10.9973, -8.5804) (11.2373, -8.4622) knots -1 -1 -1 0 0 0
  spline S696 degree 2 poles (11.2373, -8.4622) (11.4772, -8.344) (12.1743, -8.344) knots -1 -1 -1 0 0 0
  spline S697 degree 2 poles (12.1743, -8.344) (12.6494, -8.344) (12.8738, -8.3954) knots -1 -1 -1 0 0 0
  spline S698 degree 2 poles (12.8738, -8.3954) (13.0983, -8.4467) (13.2021, -8.5553) knots -1 -1 -1 0 0 0
  spline S699 degree 2 poles (13.2021, -8.5553) (13.306, -8.6639) (13.306, -8.812) knots -1 -1 -1 0 0 0
  spline S700 degree 2 poles (13.306, -8.812) (13.306, -9.0364) (13.0613, -9.1546) knots -1 -1 -1 0 0 0
  spline S701 degree 2 poles (13.0613, -9.1546) (12.8165, -9.2727) (12.1481, -9.2727) knots -1 -1 -1 0 0 0
  spline S702 degree 2 poles (13.4158, -9.9699) (13.2224, -10.0964) (12.887, -10.1668) knots 0 0 0 1 1 1
  spline S703 degree 2 poles (13.8288, -9.5234) (13.688, -9.7956) (13.4158, -9.9699) knots 0 0 0 1 1 1
  spline S704 degree 2 poles (13.9697, -8.8096) (13.9697, -9.2513) (13.8288, -9.5234) knots 0 0 0 1 1 1
  spline S705 degree 2 poles (13.528, -7.6994) (13.9697, -8.0217) (13.9697, -8.8096) knots 0 0 0 1 1 1
  spline S706 degree 2 poles (12.1337, -7.3771) (13.0863, -7.3771) (13.528, -7.6994) knots 0 0 0 1 1 1
  spline S707 degree 2 poles (11.3172, -7.475) (11.7088, -7.3771) (12.1337, -7.3771) knots 0 0 0 1 1 1
  spline S708 degree 2 poles (10.9579, -7.6075) (11.1119, -7.5251) (11.3172, -7.475) knots 0 0 0 1 1 1
  spline S709 degree 2 poles (10.6643, -7.8331) (10.8039, -7.6899) (10.9579, -7.6075) knots 0 0 0 1 1 1
  spline S710 degree 2 poles (10.4375, -8.2032) (10.5246, -7.9764) (10.6643, -7.8331) knots 0 0 0 1 1 1
  spline S711 degree 2 poles (10.3503, -8.7833) (10.3503, -8.43) (10.4375, -8.2032) knots 0 0 0 1 1 1
  spline S712 degree 2 poles (10.749, -9.878) (10.3503, -9.5186) (10.3503, -8.7833) knots 0 0 0 1 1 1
  spline S713 degree 2 poles (12.1457, -10.2373) (11.1477, -10.2373) (10.749, -9.878) knots 0 0 0 1 1 1
  spline S714 degree 2 poles (12.887, -10.1668) (12.5515, -10.2373) (12.1457, -10.2373) knots 0 0 0 1 1 1
  spline S715 degree 2 poles (2.9543, -12.1162) (2.9543, -12.2881) (3.0582, -12.3955) knots 0 0 0 1 1 1
  spline S716 degree 2 poles (3.0498, -11.8536) (2.9543, -11.9491) (2.9543, -12.1162) knots 0 0 0 1 1 1
  spline S717 degree 2 poles (3.3053, -11.7581) (3.1453, -11.7581) (3.0498, -11.8536) knots 0 0 0 1 1 1
  spline S718 degree 2 poles (3.5942, -11.8858) (3.4724, -11.7581) (3.3053, -11.7581) knots 0 0 0 1 1 1
  spline S719 degree 2 poles (3.7159, -12.2045) (3.7159, -12.0135) (3.5942, -11.8858) knots 0 0 0 1 1 1
  spline S720 degree 2 poles (3.704, -12.3311) (3.7159, -12.2499) (3.7159, -12.2045) knots 0 0 0 1 1 1
  line L211 (4.3987, -12.3812) -> (3.704, -12.3311)
  spline S721 degree 2 poles (4.3414, -12.0661) (4.3414, -12.1807) (4.3987, -12.3812) knots 0 0 0 1 1 1
  spline S722 degree 2 poles (4.4751, -11.7258) (4.3414, -11.8512) (4.3414, -12.0661) knots 0 0 0 1 1 1
  spline S723 degree 2 poles (4.8524, -11.6005) (4.6088, -11.6005) (4.4751, -11.7258) knots 0 0 0 1 1 1
  spline S724 degree 2 poles (5.2344, -11.7306) (5.0911, -11.6005) (4.8524, -11.6005) knots 0 0 0 1 1 1
  spline S725 degree 2 poles (5.3776, -12.0565) (5.3776, -11.8607) (5.2344, -11.7306) knots 0 0 0 1 1 1
  spline S726 degree 2 poles (5.2642, -12.3633) (5.3776, -12.2427) (5.3776, -12.0565) knots 0 0 0 1 1 1
  spline S727 degree 2 poles (4.8571, -12.5412) (5.1508, -12.4839) (5.2642, -12.3633) knots 0 0 0 1 1 1
  line L212 (4.9861, -13.5129) -> (4.8571, -12.5412)
  spline S728 degree 2 poles (5.5292, -13.2395) (5.3131, -13.4174) (4.9861, -13.5129) knots 0 0 0 1 1 1
  spline S729 degree 2 poles (5.8575, -12.7859) (5.7453, -13.0616) (5.5292, -13.2395) knots 0 0 0 1 1 1
  spline S730 degree 2 poles (5.9697, -12.0326) (5.9697, -12.5101) (5.8575, -12.7859) knots 0 0 0 1 1 1
  spline S731 degree 2 poles (5.8181, -11.2424) (5.9697, -11.5432) (5.9697, -12.0326) knots 0 0 0 1 1 1
  spline S732 degree 2 poles (5.386, -10.7816) (5.6665, -10.9416) (5.8181, -11.2424) knots 0 0 0 1 1 1
  spline S733 degree 2 poles (4.7998, -10.6217) (5.1054, -10.6217) (5.386, -10.7816) knots 0 0 0 1 1 1
  spline S734 degree 2 poles (4.3808, -10.7183) (4.5563, -10.6217) (4.7998, -10.6217) knots 0 0 0 1 1 1
  spline S735 degree 2 poles (4.0979, -10.9893) (4.2054, -10.815) (4.3808, -10.7183) knots 0 0 0 1 1 1
  spline S736 degree 2 poles (3.9809, -11.2997) (4.0311, -11.0968) (4.0979, -10.9893) knots 0 0 0 1 1 1
  spline S737 degree 2 poles (3.6586, -10.9249) (3.8425, -11.049) (3.9809, -11.2997) knots 0 0 0 1 1 1
  spline S738 degree 2 poles (3.248, -10.8007) (3.4748, -10.8007) (3.6586, -10.9249) knots 0 0 0 1 1 1
  spline S739 degree 2 poles (2.6058, -11.1063) (2.8612, -10.8007) (3.248, -10.8007) knots 0 0 0 1 1 1
  spline S740 degree 2 poles (2.3503, -12.0971) (2.3503, -11.4119) (2.6058, -11.1063) knots 0 0 0 1 1 1
  spline S741 degree 2 poles (2.5843, -13.0198) (2.3503, -12.694) (2.3503, -12.0971) knots 0 0 0 1 1 1
  spline S742 degree 2 poles (3.2575, -13.4603) (2.8183, -13.3457) (2.5843, -13.0198) knots 0 0 0 1 1 1
  line L213 (3.4223, -12.5412) -> (3.2575, -13.4603)
  spline S743 degree 2 poles (3.0582, -12.3955) (3.162, -12.503) (3.4223, -12.5412) knots 0 0 0 1 1 1
  spline S744 degree 2 poles (-7.8519, -9.2727) (-8.5133, -9.2727) (-8.758, -9.1653) knots -1 -1 -1 0 0 0
  spline S745 degree 2 poles (-8.758, -9.1653) (-9.0027, -9.0579) (-9.0027, -8.8167) knots -1 -1 -1 0 0 0
  spline S746 degree 2 poles (-9.0027, -8.8167) (-9.0027, -8.5804) (-8.7627, -8.4622) knots -1 -1 -1 0 0 0
  spline S747 degree 2 poles (-8.7627, -8.4622) (-8.5228, -8.344) (-7.8257, -8.344) knots -1 -1 -1 0 0 0
  spline S748 degree 2 poles (-7.8257, -8.344) (-7.3506, -8.344) (-7.1262, -8.3954) knots -1 -1 -1 0 0 0
  spline S749 degree 2 poles (-7.1262, -8.3954) (-6.9017, -8.4467) (-6.7979, -8.5553) knots -1 -1 -1 0 0 0
  spline S750 degree 2 poles (-6.7979, -8.5553) (-6.694, -8.6639) (-6.694, -8.812) knots -1 -1 -1 0 0 0
  spline S751 degree 2 poles (-6.694, -8.812) (-6.694, -9.0364) (-6.9387, -9.1546) knots -1 -1 -1 0 0 0
  spline S752 degree 2 poles (-6.9387, -9.1546) (-7.1835, -9.2727) (-7.8519, -9.2727) knots -1 -1 -1 0 0 0
  spline S753 degree 2 poles (-6.5842, -9.9699) (-6.7776, -10.0964) (-7.113, -10.1668) knots 0 0 0 1 1 1
  spline S754 degree 2 poles (-6.1712, -9.5234) (-6.312, -9.7956) (-6.5842, -9.9699) knots 0 0 0 1 1 1
  spline S755 degree 2 poles (-6.0303, -8.8096) (-6.0303, -9.2513) (-6.1712, -9.5234) knots 0 0 0 1 1 1
  spline S756 degree 2 poles (-6.472, -7.6994) (-6.0303, -8.0217) (-6.0303, -8.8096) knots 0 0 0 1 1 1
  spline S757 degree 2 poles (-7.8663, -7.3771) (-6.9137, -7.3771) (-6.472, -7.6994) knots 0 0 0 1 1 1
  spline S758 degree 2 poles (-8.6828, -7.475) (-8.2912, -7.3771) (-7.8663, -7.3771) knots 0 0 0 1 1 1
  spline S759 degree 2 poles (-9.0421, -7.6075) (-8.8881, -7.5251) (-8.6828, -7.475) knots 0 0 0 1 1 1
  spline S760 degree 2 poles (-9.3357, -7.8331) (-9.1961, -7.6899) (-9.0421, -7.6075) knots 0 0 0 1 1 1
  spline S761 degree 2 poles (-9.5625, -8.2032) (-9.4754, -7.9764) (-9.3357, -7.8331) knots 0 0 0 1 1 1
  spline S762 degree 2 poles (-9.6497, -8.7833) (-9.6497, -8.43) (-9.5625, -8.2032) knots 0 0 0 1 1 1
  spline S763 degree 2 poles (-9.251, -9.878) (-9.6497, -9.5186) (-9.6497, -8.7833) knots 0 0 0 1 1 1
  spline S764 degree 2 poles (-7.8543, -10.2373) (-8.8523, -10.2373) (-9.251, -9.878) knots 0 0 0 1 1 1
  spline S765 degree 2 poles (-7.113, -10.1668) (-7.4485, -10.2373) (-7.8543, -10.2373) knots 0 0 0 1 1 1
  line L214 (20.5014, -11.8273) -> (20.5014, -12.7633)
  line L215 (20.5014, -12.7633) -> (19.3999, -11.8273)
  line L216 (19.3999, -11.8273) -> (20.5014, -11.8273)
  line L217 (21.91, -10.9798) -> (21.91, -11.8273)
  line L218 (21.2558, -10.9798) -> (21.91, -10.9798)
  line L219 (21.2558, -10.5405) -> (21.2558, -10.9798)
  line L220 (20.5014, -10.5405) -> (21.2558, -10.5405)
  line L221 (20.5014, -10.9798) -> (20.5014, -10.5405)
  line L222 (18.3503, -10.9798) -> (20.5014, -10.9798)
  line L223 (18.3503, -11.8273) -> (18.3503, -10.9798)
  line L224 (20.456, -13.5988) -> (18.3503, -11.8273)
  line L225 (21.2558, -13.5988) -> (20.456, -13.5988)
  line L226 (21.2558, -11.8273) -> (21.2558, -13.5988)
  line L227 (21.91, -11.8273) -> (21.2558, -11.8273)